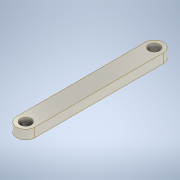
# Autodesk Inventor part: Pieza1
Saved by Autodesk Inventor 2021 (Build 250183000, 183)
## iProperties
Created: 2021-07-30
Part Number: Pieza1
Material: Titanio
Document SubType Name: Modeling
Designer: uriel
Density: 4.51 g/cm^3
Appearance: Titanio
Author: uriel
Autodesk Inventor part; units mm, degrees
ref_plane "YZ Plane" through (0, 0, 0) normal (1, 0, 0) x (0, 1, 0)
ref_plane "XZ Plane" through (0, 0, 0) normal (0, 1, 0) x (-1, 0, 0)
ref_plane "XY Plane" through (0, 0, 0) normal (0, 0, 1) x (1, 0, 0)
sketch "Boceto1" plane through (0, 0, 0) normal (0, 1, 0) x (-1, 0, 0)
  line L0 (5, 40) -> (-5, 40)
  line L1 (-5, 40) -> (-5, -40)
  line L2 (-5, -40) -> (5, -40)
  line L3 (5, -40) -> (5, 40)
  line L4 (5, 40) -> (-5, -40) construction
  line L5 (-5, 40) -> (5, -40) construction
  circle A0 centre (0, 35) radius 3
  circle A1 centre (0, -35) radius 3
  point P0 (0, 0)
  dimension "d0" = 10
  dimension "d1" = 80
  dimension "d2" = 6
  dimension "d3" = 6
  dimension "d4" = 5
  dimension "d5" = 5
  constraints: 12 end point, 2 centre point, 2 midpoint, 2 parallel, 1 horizontal, 1 perpendicular
  measures "d0" distance of L2.end L1.end
  measures "d1" distance of L1.end L0.end
  measures "d2" diameter of A0
  measures "d3" diameter of A1
  measures "d4" distance from line of L2 A1.centre
  measures "d5" distance from line of L0 A0.centre
extrude "Extrusión1" add sketch "Boceto1" along normal mid plane 5
fillet "Empalme1" radius 5 4 edges at (-5, 0, 40) (5, 0, 40) (5, 0, -40) (-5, 0, -40)
